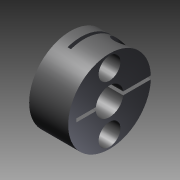
# Autodesk Inventor part: SSTHMR12b
Saved by Autodesk Inventor 2011 SP1 (Build 150282100, 282)
## iProperties
Created: 2016-04-05
Part Number: SSTHMR12b
Catalog Web Link: www.cadenas.de
Description: STHMRB, STHMR, SSTHMR-b-Shaft Supports - Bracket Shaped Compact - Standard Type
Vendor: MISUMI
Document SubType Name: Modeling
Designer: psAdmin
Manufacturer: MISUMI
Mass: 11.7065 g
Surface Area: 64.9723 cm^2
Volume: 11.7065 cm^3
Density: 1 g/cm^3
Category: PARTsolutions
Company: MISUMI
Title: SSTHMR12b
Author: Cadenas PARTsolutions
Comments: Shaft Supports - Bracket Shaped Compact - Standard Type
PSOL_IDENT_0: {$CADENAS_DATA\23d-libs\misumi\metric\02_shaft_supports\sthmrb_b.prj},183 {VTYP=3D},{NB=SSTHMR12b},{
PSOL_IDENT_1: LINA=SSTHMR12b},{NN=STHMRB, STHMR, SSTHMR-b},{DATE=21.05.2015 05:05:32},{GEOMDATE=21.05.2015 05:05:3
PSOL_IDENT_2: 2},{VERSION=},{LINEID=70},{LINESUBID=-1},{WBVAR=MAT,ST}  {NB=SSTHMR12b},{LINA=SSTHMR12b},{KT=DUMMY},
PSOL_IDENT_3: {PN=SSTHMR12},{TYPE=SSTHMR},{MAT=SUS304},{ST=-},{AC=Hexagon Socket Head Cap Screw (1 Pc.) (304 Stain
PSOL_IDENT_4: less Steel) },{D=12},{DH=12},{L=17},{H=36},{B=11},{T=4.5},{P=25},{DD1=5.5},{DD2=9.5},{S=1.5},{X=12.0
PSOL_IDENT_5: },{Y=6},{M=5},{DD=5.5},{R=9},{THMD=5},{ST0='-','-'},{BOLT=M5x12},{LL=12},{COL=0.75,0.75,0.75,0.00}
NN: STHMRB, STHMR, SSTHMR-b
NT: Shaft Supports - Bracket Shaped Compact - Standard Type
NB: SSTHMR12b
NBSYN: $PN.b
LINA: SSTHMR12b
PN: SSTHMR12
MAT: SUS304
ST: -
AC: Hexagon Socket Head Cap Screw (1 Pc.) (304 Stainless Steel)
D: 12
DH: 12
L: 17
H: 36
B: 11
T: 4.5
P: 25
DD1: 5.5
DD2: 9.5
S: 1.5
X: 12.0
Y: 6
M: 5
DD: 5.5
R: 9
THMD: 5
BOLT: M5x12
LL: 12
SUPPLIER: MISUMI
ARTICLENO: SSTHMR12b
BOMINFO: SSTHMR12b
CREATOR: CADENAS GmbH
Autodesk Inventor part; units mm, degrees
sketch "Sketch_1" plane through (0, 0, 0) normal (0, 0, 1) x (1, 0, 0)
  line L0 (17, 0) -> (0, 0)
  line L1 (0, 18) -> (0, 6)
  line L2 (0, 6) -> (17, 6)
  line L3 (17, 6) -> (17, 18)
  line L4 (17, 18) -> (0, 18)
  constraints: 10 end point
revolve "Revolution1" add sketch "Sketch_1" angle 360 about axis through (17, 0, 0) along (1, 0, 0)
sketch "Sketch_2" plane through (0, 0, 0) normal (0, 0, 1) x (1, 0, 0)
  line L0 (4.5, -5.8) -> (6, -5.8)
  line L1 (6, -5.8) -> (6, 30.2)
  line L2 (6, 30.2) -> (4.5, 30.2)
  line L3 (4.5, 30.2) -> (4.5, -5.8)
  constraints: 8 end point
extrude "Extrusion1" cut sketch "Sketch_2" along normal mid plane 36
sketch "Sketch3" plane through (17, 0, 0) normal (1, 0, 0) x (0, 0, -1)
  point P0 (-12.5, 0)
hole "Hole1" at (17, 0, 12.5) direction (-1, 0, 0) diameter 5.5 depth 17 counterbore diameter 9.5 counterbore depth 12.5
sketch "Sketch4" plane through (17, 0, 0) normal (1, 0, 0) x (0, 0, -1)
  point P0 (12.5, 0)
hole "Hole2" at (17, 0, -12.5) direction (-1, 0, 0) diameter 5.5 depth 17 counterbore diameter 9.5 counterbore depth 12.5
sketch "Sketch_5" plane through (17, 0, 0) normal (1, 0, 0) x (0, 0, -1)
  line L0 (-0.75, 0) -> (0.75, 0)
  line L1 (0.75, 0) -> (0.75, 36)
  line L2 (0.75, 36) -> (-0.75, 36)
  line L3 (-0.75, 36) -> (-0.75, 0)
  constraints: 8 end point
extrude "Extrusion2" cut sketch "Sketch_5" against normal blind 11
sketch "Sketch_6" plane through (0, 0, 0) normal (0, 0, 1) x (1, 0, 0)
  arc A0 (9.5, -6) -> (17, -14.4) centre (26.2631, 1.4189) ccw
  line L0 (17, -14.4) -> (17, 3.6)
  line L1 (17, 3.6) -> (9.5, 3.6)
  line L2 (9.5, 3.6) -> (9.5, -6)
  constraints: 6 end point, 2 point on circle, 1 centre point
extrude "Extrusion3" cut sketch "Sketch_6" along normal mid plane 1.5
sketch "Sketch_4" plane through (11.5, 0, 0) normal (1, 0, 0) x (0, 0, -1)
  line L0 (0, 12) -> (-18, 12)
  line L1 (-18, 12) -> (-18, 16.5)
  line L2 (-18, 16.5) -> (-6, 16.5)
  line L3 (-6, 16.5) -> (-6, 14.75)
  line L4 (-6, 14.75) -> (0, 14.75)
  line L5 (0, 14.75) -> (0, 12)
  line L6 (0, 12) -> (-18, 12)
  constraints: 14 end point
revolve "Revolution2" cut sketch "Sketch_4" angle 360 about axis through (11.5, 12, 0) along (0, 0, -1)
sketch "Sketch_7" plane through (11.5, 0, 0) normal (1, 0, 0) x (0, 0, -1)
  line L0 (0.75, 12) -> (15.2889, 12)
  line L1 (15.2889, 12) -> (15.2889, 9.5)
  line L2 (15.2889, 9.5) -> (14.8559, 9.933)
  line L3 (14.8559, 9.933) -> (1.183, 9.933)
  line L4 (1.183, 9.933) -> (0.75, 9.5)
  line L5 (0.75, 9.5) -> (0.75, 12)
  line L6 (0.75, 12) -> (15.2889, 12)
  constraints: 14 end point
revolve "Revolution3" cut sketch "Sketch_7" angle 360 about axis through (11.5, 12, -0.75) along (0, 0, 1)
thread "Thread1" size "M5x0.8" class "6H" standard "ISO Metric profile" length 13.6729
ref_plane "b_s_XY" through (11.5, 12, 6) normal (0, 0, 1) x (1, 0, 0)
ref_plane "b_s_YZ" through (11.5, 12, 6) normal (1, 0, 0) x (0, 1, 0)
ref_plane "b_s_ZX" through (11.5, 12, 6) normal (0, 1, 0) x (0, 0, 1)
body "Solid1"
